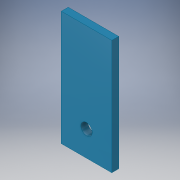
# Autodesk Inventor part: IRBoard
Saved by Autodesk Inventor 2018 (Build 220112000, 112)
## iProperties
Created: 2018-01-13
Part Number: IRBoard
Material: Thermoplastic Resin
Document SubType Name: Modeling
Designer: Kyle-HP
Density: 1.28 g/cm^3
Appearance: Sky Blue Dark
Author: Kyle-HP
Autodesk Inventor part; units mm, degrees
ref_plane "YZ Plane" through (0, 0, 0) normal (1, 0, 0) x (0, 1, 0)
ref_plane "XZ Plane" through (0, 0, 0) normal (0, 1, 0) x (-1, 0, 0)
ref_plane "XY Plane" through (0, 0, 0) normal (0, 0, 1) x (1, 0, 0)
sketch "Sketch1" plane through (0, 0, 0) normal (0, 0, 1) x (1, 0, 0)
  line L0 (0, 0) -> (13.97, 0)
  line L1 (13.97, 0) -> (13.97, -31.75)
  line L2 (13.97, -31.75) -> (0, -31.75)
  line L3 (0, -31.75) -> (0, 0)
  dimension "d0" = 13.97
  dimension "d1" = 31.75
  constraints: 8 end point, 2 parallel, 1 horizontal, 1 perpendicular
  measures "d0" distance of L0.start L0.end
  measures "d1" distance of L0.end L1.end
extrude "Extrusion1" add sketch "Sketch1" along normal blind 1.905
sketch "Sketch2" plane through (0, 0, 1.905) normal (0, 0, 1) x (1, 0, 0)
  circle A0 centre (6.985, -24.765) radius 1.5875
  line L0 (13.97, -31.75) -> (13.97, 0) projected
  line L1 (0, -31.75) -> (13.97, -31.75) projected
  point P0 (0, 0)
  dimension "d4" = 3.175
  dimension "d5" = 6.985
  dimension "d6" = 6.985
  constraints: 1 centre point
  measures "d4" diameter of A0
  measures "d5" distance from line of A0.centre L0
  measures "d6" distance from line of A0.centre L1
extrude "Extrusion2" cut sketch "Sketch2" against normal blind 1.905
body "Solid1"
